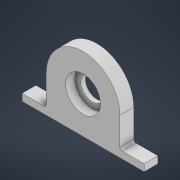
# Autodesk Inventor part: Halterung_Differential_Mitte
Saved by Autodesk Inventor 2021 (Build 250183000, 183)
## iProperties
Created: 2021-01-29
Part Number: Halterung_Differential_Mitte
Material: Generisch
Document SubType Name: Modeling
Designer: laure
Density: 1 g/cm^3
Appearance: Vorgabe
Author: laure
Autodesk Inventor part; units mm, degrees
ref_plane "YZ Plane" through (0, 0, 0) normal (1, 0, 0) x (0, 1, 0)
ref_plane "XZ Plane" through (0, 0, 0) normal (0, 1, 0) x (-1, 0, 0)
ref_plane "XY Plane" through (0, 0, 0) normal (0, 0, 1) x (1, 0, 0)
sketch "Skizze1" plane through (0, 0, 0) normal (0, 0, 1) x (1, 0, 0)
  line L0 (-16, 16) -> (16, 16)
  line L1 (16, 16) -> (16, -16)
  line L2 (16, -16) -> (-16, -16)
  line L3 (-16, -16) -> (-16, 16)
  line L4 (0, 22.4) -> (0, -22.4) projected
  line L5 (-22.4, 0) -> (22.4, 0) projected
  point P0 (0, 0)
  dimension "d0" = 32
  dimension "d1" = 32
  constraints: 8 end point, 2 parallel, 1 horizontal, 1 perpendicular, 2 other
  measures "d0" distance of L0.start L0.end
  measures "d1" distance of L0.end L1.end
extrude "Extrusion1" add sketch "Skizze1" along normal mid plane 6
sketch "Skizze2" plane through (0, 0, 0) normal (0, 0, 1) x (1, 0, 0)
  line L0 (-16, 16) -> (-16, -16) projected
  line L1 (-16, -16) -> (-26.5, -16)
  line L2 (-26.5, -16) -> (-26.5, -13)
  line L3 (-26.5, -13) -> (-16, -13)
  line L4 (-16, -13) -> (-16, -16)
  line L5 (0, 22.4) -> (0, -22.4) projected
  line L6 (16, -16) -> (26.5, -16)
  line L7 (26.5, -16) -> (26.5, -13)
  line L8 (26.5, -13) -> (16, -13)
  line L9 (16, -13) -> (16, -16)
  point P0 (0, 0)
  dimension "d6" = 10.5
  dimension "d7" = 3
  constraints: 16 end point, 4 symmetric about line, 2 parallel, 1 horizontal, 1 perpendicular
  measures "d6" distance of L2.end L3.end
  measures "d7" distance between parallel lines of L1 L3
extrude "Extrusion2" add sketch "Skizze2" along normal mid plane 6
fillet "Rundung1" radius 16 2 edges at (-16, 16, 0) (16, 16, 0)
fillet "Rundung2" radius 1 2 edges at (-16, -13, 0) (16, -13, 0)
sketch "Skizze3" plane through (0, 0, 3) normal (0, 0, 1) x (1, 0, 0)
  circle A0 centre (0, 0) radius 7.6
  dimension "d12" = 15.2
  constraints: 1 centre point, 1 coincident
  measures "d12" diameter of A0
extrude "Extrusion3" cut sketch "Skizze3" against normal blind 4
sketch "Skizze4" plane through (0, 0, -1) normal (0, 0, 1) x (1, 0, 0)
  circle A0 centre (0, 0) radius 5
  dimension "d15" = 10
  constraints: 1 centre point, 1 coincident
  measures "d15" diameter of A0
extrude "Extrusion4" cut sketch "Skizze4" against normal up to surface (2 mm away)
